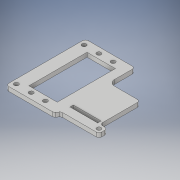
# Autodesk Inventor part: coxaa
Saved by Autodesk Inventor 2019 (Build 230136000, 136)
## iProperties
Created: 2023-04-15
Part Number: coxaa
Material: Generic
Document SubType Name: Modeling
Designer: Analuam
Density: 1 g/cm^3
Appearance: Default
Author: Analuam
Autodesk Inventor part; units mm, degrees
ref_plane "YZ Plane" through (0, 0, 0) normal (1, 0, 0) x (0, 1, 0)
ref_plane "XZ Plane" through (0, 0, 0) normal (0, 1, 0) x (-1, 0, 0)
ref_plane "XY Plane" through (0, 0, 0) normal (0, 0, 1) x (1, 0, 0)
sketch "Sketch1" plane through (0, 0, 0) normal (0, 1, 0) x (-1, 0, 0)
  line L0 (10.5532, 14.1338) -> (-9.4468, 14.1338)
  line L1 (-9.4468, 14.1338) -> (-9.4468, -26.8662)
  line L2 (-9.4468, -26.8662) -> (10.5532, -26.8662)
  line L3 (10.5532, -26.8662) -> (10.5532, 14.1338)
  circle A0 centre (5.5532, 17.5338) radius 1.5
  line L4 (19.2289, 19.6338) -> (19.2289, -32.3662)
  line L5 (17.2289, -34.3662) -> (-13.7711, -34.3662)
  line L6 (-15.7711, -32.3662) -> (-15.7711, -19.826)
  line L7 (-19.7711, -15.826) -> (-35.887, -15.826)
  line L8 (-37.887, -13.826) -> (-37.887, 10.574)
  line L9 (17.2289, 21.6338) -> (-13.3861, 21.6338)
  line L10 (-14.943, 20.8893) -> (-16.2097, 19.3185)
  line L11 (-17.7665, 18.574) -> (-35.887, 18.574)
  line L12 (-16.8101, 12.574) -> (-36.4101, 12.574)
  line L13 (-36.4101, 12.574) -> (-36.4101, 10.174)
  line L14 (-36.4101, 10.174) -> (-16.8101, 10.174)
  line L15 (-16.8101, 10.174) -> (-16.8101, 12.574)
  circle A1 centre (-4.4468, 17.5338) radius 1.5
  circle A2 centre (5.5532, -30.2662) radius 1.5
  circle A3 centre (-4.4468, -30.2662) radius 1.5
  arc A4 (19.2289, 19.6338) -> (17.2289, 21.6338) centre (17.2289, 19.6338) ccw
  arc A5 (17.2289, -34.3662) -> (19.2289, -32.3662) centre (17.2289, -32.3662) ccw
  arc A6 (-15.7711, -32.3662) -> (-13.7711, -34.3662) centre (-13.7711, -32.3662) ccw
  arc A7 (-15.7711, -19.826) -> (-19.7711, -15.826) centre (-19.7711, -19.826) ccw
  arc A8 (-37.887, -13.826) -> (-35.887, -15.826) centre (-35.887, -13.826) ccw
  arc A9 (-17.7665, 18.574) -> (-16.2097, 19.3185) centre (-17.7665, 20.574) ccw
  arc A10 (-13.3861, 21.6338) -> (-14.943, 20.8893) centre (-13.3861, 19.6338) ccw
  line L16 (-33.327, 18.574) -> (-41.327, 18.574)
  line L17 (-43.327, 16.574) -> (-43.327, 14.574)
  line L18 (-41.327, 12.574) -> (-39.887, 12.574)
  circle A11 centre (-40.327, 15.574) radius 1.5
  arc A12 (-37.887, 10.574) -> (-39.887, 12.574) centre (-39.887, 10.574) ccw
  arc A13 (-43.327, 14.574) -> (-41.327, 12.574) centre (-41.327, 14.574) ccw
  arc A14 (-41.327, 18.574) -> (-43.327, 16.574) centre (-41.327, 16.574) ccw
  circle A15 centre (16.0065, 17.5338) radius 1.5
  circle A16 centre (16.0065, -30.2662) radius 1.5
  point P0 (0, 0)
  point P1 (-43.327, 12.574)
  dimension "d0" = 20
  dimension "d1" = 41
  dimension "d2" = 3
  dimension "d3" = 3.4
  dimension "d5" = 19.6
  dimension "d6" = 2.4
  dimension "d7" = 26
  dimension "d8" = 6
  dimension "d9" = 56
  dimension "d10" = 7.5
  dimension "d11" = 2
  dimension "d12" = 4
  dimension "d14" = 3
  dimension "d15" = 2
  dimension "d16" = 3
  dimension "d17" = 35
  dimension "d18" = 3
  constraints: 38 end point, 20 point on circle, 20 tangent, 17 centre point, 8 perpendicular, 7 equal radius, 5 parallel, 4 horizontal, 3 point on line, 1 vertical
  measures "d0" distance of L2.end L1.end
  measures "d1" distance of L1.end L0.end
  measures "d2" diameter of A0
  measures "d3" distance from line of L0 A0.centre
  measures "d5" distance of L14.end L13.end
  measures "d6" distance of L13.end L12.end
  measures "d7" distance between parallel lines of L7 L14
  measures "d8" distance between parallel lines of L11 L12
  measures "d9" distance between parallel lines of L5 L9
  measures "d10" distance between parallel lines of L9 L0
  measures "d11" radius of A4
  measures "d12" radius of A7
  measures "d14" diameter of A11
  measures "d15" radius of A12
  measures "d16" distance from line of L17 A11.centre
  measures "d17" distance between parallel lines of L4 L6
  measures "d18" diameter of A15
extrude "Extrusion1" add sketch "Sketch1" along normal blind 3
body "Solid1"
